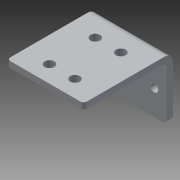
# Autodesk Inventor part: Pneumatic Piston Back Flange (Custom)
Saved by Autodesk Inventor 2014 (Build 180170000, 170)
## iProperties
Created: 2014-01-17
Part Number: Pneumatic Piston Back Flange (Custom)
Material: Aluminum 6061
Document SubType Name: Sheet Metal
Designer: Michael
Density: 2.71 g/cm^3
Sheet Metal Rule: Default
Appearance: Aluminum - Flat
Author: Michael
Autodesk Inventor part; units mm, degrees
ref_plane "YZ Plane" through (0, 0, 0) normal (1, 0, 0) x (0, 1, 0)
ref_plane "XZ Plane" through (0, 0, 0) normal (0, 1, 0) x (-1, 0, 0)
ref_plane "XY Plane" through (0, 0, 0) normal (0, 0, 1) x (1, 0, 0)
sketch "Sketch1" plane through (0, 0, 0) normal (0, 0, 1) x (1, 0, 0)
  line L0 (0, 0) -> (38.1, 0)
  line L1 (38.1, 0) -> (38.1, 25.4)
  line L2 (38.1, 25.4) -> (0, 25.4)
  line L3 (0, 25.4) -> (0, 0)
  circle A0 centre (6.35, 12.7) radius 2.0701
  line L4 (0, 12.7) -> (38.1, 12.7) construction
  circle A1 centre (31.75, 12.7) radius 2.0701
  dimension "d0" = 38.1
  dimension "d1" = 25.4
  dimension "d2" = 4.1402
  dimension "d3" = 6.35
  dimension "d6" = 25.4
  measures "d0" distance of L2.end L1.end
  measures "d1" distance of L1.end L0.end
  measures "d2" diameter of A0
  measures "d3" distance from line of L3 A0.centre
  measures "d6" distance of A0.centre A1.centre
extrude "Plate1" add sketch "Sketch1" along normal blind 3.048
sketch "Sketch2" plane through (0, 26.67, 4.318) normal (0, 1, 0) x (-1, 0, 0)
  line L0 (-38.1, 0) -> (0, 0)
  line L1 (0, 0) -> (0, 40.132)
  line L2 (0, 40.132) -> (-38.1, 40.132)
  line L3 (-38.1, 40.132) -> (-38.1, 0)
  constraints: 6 end point, 1 horizontal, 1 perpendicular, 1 vertical
edge flange "Flange1" height 44.45 angle 90 thickness 3.048 bend radius 1.27 thickness toward (0, 1, 0) relief straight relief width 3.048 relief depth 1.524 edges at (19.05, 25.4, 3.048) wall of the first edge with corners at (38.1, 26.67, 4.318) (0, 26.67, 4.318) (0, 26.67, 44.45) (38.1, 26.67, 44.45)
bend "Bend1"
corner "Corner1"
fillet "Fillet1" radius 1.5875 4 edges at (38.1, 0, 1.524) (0, 0, 1.524) (0, 28.194, 44.45) (38.1, 28.194, 44.45)
sketch "Sketch3" plane through (0, 26.67, 4.318) normal (0, -1, 0) x (1, 0, 0)
  line L0 (0, 38.5445) -> (0, 0) projected
  line L1 (0, 0) -> (38.1, 0) projected
  line L2 (9.525, 37.465) -> (28.575, 37.465) construction
  line L3 (28.575, 37.465) -> (28.575, 3.175) construction
  line L4 (28.575, 3.175) -> (9.525, 3.175) construction
  line L5 (9.525, 3.175) -> (9.525, 37.465) construction
  circle A0 centre (25.4, 31.7119) radius 2.413
  line L6 (19.05, 37.465) -> (19.05, 3.175) construction
  line L7 (9.525, 20.32) -> (28.575, 20.32) construction
  circle A1 centre (12.7, 31.7119) radius 2.413
  circle A2 centre (25.4, 8.9281) radius 2.413
  circle A3 centre (12.7, 8.9281) radius 2.413
  point P0 (0, -4.318)
  dimension "d23" = 34.29
  dimension "d24" = 19.05
  dimension "d25" = 3.175
  dimension "d26" = 9.525
  dimension "d27" = 4.826
  dimension "d28" = 3.175
  dimension "d29" = 5.7531
  constraints: 12 end point, 4 centre point, 4 midpoint, 3 symmetric about line, 2 parallel, 1 horizontal, 1 perpendicular, 3 other
  measures "d23" distance of L4.end L2.start
  measures "d24" distance of L2.start L2.end
  measures "d25" distance between parallel lines of L1 L4
  measures "d26" distance between parallel lines of L0 L5
  measures "d27" diameter of A0
  measures "d28" distance from line of L3 A0.centre
  measures "d29" distance from line of A0.centre L2
extrude "Extrusion1" cut sketch "Sketch3" against normal blind 25.4
equation "\"d12\" = BendReliefWidth"
equation "\"d13\" = BendReliefDepth"
equation "\"d14\" = MinimumRemnant"
equation "\"d15\" = BendRadius"
equation "\"d19\" = CornerReliefSize"
equation "\"d20\" = GapSize"
equation "\"d21\" = JacobiRadiusSize"
equation "\"BendRadius\" = Thickness"
equation "\"BendReliefWidth\" = Thickness"
equation "\"BendReliefDepth\" = 0.5 * Thickness"
equation "\"CornerReliefSize\" = 4 * Thickness"
equation "\"MinimumRemnant\" = 2 * Thickness"
equation "\"TransitionRadius\" = BendRadius"
equation "\"JacobiRadiusSize\" = BendRadius"
equation "\"GapSize\" = Thickness"
equation "\"d11\" = BendRadius"
equation "\"Thickness\" = 3.048"
body "Solid1"
